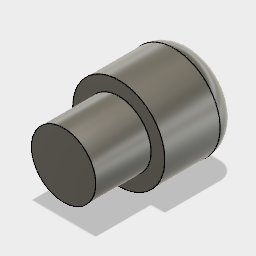
Temp_Buttom_New (Autodesk Fusion 360 design; units mm, degrees)
Autodesk Fusion 360 part; units mm, degrees
sketch "Sketch1" plane through (0, 0, 0) normal (0, 0, 1) x (1, 0, 0)
  circle A0 centre (0, 0) radius 2.5
  circle A1 centre (0, 0) radius 1.75
  dimension "d1" = 5
  dimension "d2" = 3.5
  measures "d1" diameter of A0
  measures "d2" diameter of A1
extrude "Extrude1" add sketch "Sketch1" along normal blind 4 contours A0 | A1
extrude "Extrude2" add sketch "Sketch1" along normal blind 7 contours A1
fillet "Fillet1" radius 1 1 edges at (-2.3308, -0.904, 0)
